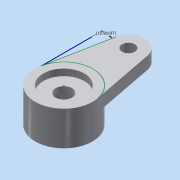
# Autodesk Inventor part: ServoHorn10mmPitch
Saved by Autodesk Inventor 2017 (Build 210142000, 142)
## iProperties
Created: 2016-11-02
Part Number: ServoHorn10mmPitch
Material: ABS Plastic
Document SubType Name: Modeling
Designer: techn
Density: 1.06 g/cm^3
Appearance: Smooth - White
Author: techn
Autodesk Inventor part; units mm, degrees
ref_plane "YZ Plane" through (0, 0, 0) normal (1, 0, 0) x (0, 1, 0)
ref_plane "XZ Plane" through (0, 0, 0) normal (0, 1, 0) x (-1, 0, 0)
ref_plane "XY Plane" through (0, 0, 0) normal (0, 0, 1) x (1, 0, 0)
sketch "Sketch1" plane through (0, 0, 0) normal (0, 1, 0) x (-1, 0, 0)
  circle A0 centre (0, 0) radius 2.8702
  dimension "d0" = 5.7404
  constraints: 1 centre point, 1 coincident
  measures "d0" diameter of A0
extrude "Extrusion1" add sketch "Sketch1" along normal blind 3.4036
sketch "Sketch2" plane through (0, 3.4036, 0) normal (0, 1, 0) x (1, 0, 0)
  circle A0 centre (0, 0) radius 4.445
  line L0 (0, 0) -> (0, 10)
  circle A1 centre (0, 10) radius 1
  circle A2 centre (0, 10) radius 2.54
  line L1 (-4.3636, 0.8468) -> (-2.4935, 10.4839)
  line L2 (4.3636, 0.8468) -> (2.4935, 10.4839)
  dimension "d3" = 8.89
  dimension "d4" = 10
  dimension "d5" = 2
  dimension "d6" = 5.08
  constraints: 6 end point, 4 point on circle, 4 tangent, 3 centre point, 3 coincident, 1 vertical
  measures "d3" diameter of A0
  measures "d4" distance of L0.start L0.end
  measures "d5" diameter of A1
  measures "d6" diameter of A2
extrude "Extrusion2" add sketch "Sketch2" along normal blind 1.905
sketch "Sketch3" plane through (0, 5.3086, 0) normal (0, 1, 0) x (1, 0, 0)
  circle A0 centre (0, 0) radius 1.27
  dimension "d9" = 2.54
  constraints: 1 centre point, 1 coincident
  measures "d9" diameter of A0
extrude "Extrusion3" cut sketch "Sketch3" against normal through all
sketch "Sketch4" plane through (0, 5.3086, 0) normal (0, 1, 0) x (1, 0, 0)
  circle A0 centre (0, 0) radius 3.175
  dimension "d12" = 6.35
  constraints: 1 centre point, 1 coincident
  measures "d12" diameter of A0
extrude "Extrusion4" cut sketch "Sketch4" against normal blind 1.016
sketch "Sketch5" plane through (0, 0, 0) normal (0, -1, 0) x (1, 0, 0)
  circle A0 centre (0, 0) radius 4.445
  circle A1 centre (0, 0) radius 2.8702 projected
  arc A2 (4.3636, -0.8468) -> (-4.3636, -0.8468) centre (0, 0) ccw projected
  dimension "d21" = 8.89
  constraints: 1 centre point, 1 coincident
  measures "d21" diameter of A0
extrude "Extrusion6" add sketch "Sketch5" against normal up to surface (3.4036 mm away)
extrude "Extrusion7" cut sketch "Sketch5" against normal blind 3.4036 contours A1
body "Solid1"
